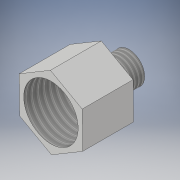
# Autodesk Inventor part: adapter
Saved by Autodesk Inventor 2018 (Build 220112000, 112)
## iProperties
Created: 2017-05-02
Part Number: adapter
Material: Generic
Document SubType Name: Modeling
Designer: gsegs
Density: 1 g/cm^3
Appearance: Default
Author: gsegs
Autodesk Inventor part; units mm, degrees
ref_plane "YZ Plane" through (0, 0, 0) normal (1, 0, 0) x (0, 1, 0)
ref_plane "XZ Plane" through (0, 0, 0) normal (0, 1, 0) x (-1, 0, 0)
ref_plane "XY Plane" through (0, 0, 0) normal (0, 0, 1) x (1, 0, 0)
sketch "Sketch1" plane through (0, 0, 0) normal (0, 0, 1) x (1, 0, 0)
  line L0 (21.8129, 13.019) -> (22.1812, -12.381)
  line L1 (22.1812, -12.381) -> (0.3684, -25.4)
  line L2 (0.3684, -25.4) -> (-21.8129, -13.019)
  line L3 (-21.8129, -13.019) -> (-22.1812, 12.381)
  line L4 (-22.1812, 12.381) -> (-0.3684, 25.4)
  line L5 (-0.3684, 25.4) -> (21.8129, 13.019)
  point P0 (0, 0)
  point P1 (0, 0)
  dimension "d0" = 25.4
  dimension "d1" = 120
  constraints: 12 end point, 1 coincident, 13 other
  measures "d0" vertical distance of L2.end L3.end
  measures "d1" angle of L2 L3
extrude "Extrusion1" add sketch "Sketch1" along normal blind 35.56
sketch "Sketch2" plane through (0, 0, 35.56) normal (0, 0, 1) x (1, 0, 0)
  circle A0 centre (0, 0) radius 19.05
  dimension "d4" = 38.1
  constraints: 1 centre point, 1 coincident
  measures "d4" diameter of A0
extrude "Extrusion2" cut sketch "Sketch2" against normal blind 30.48
sketch "Sketch3" plane through (0, 0, 0) normal (0, 0, -1) x (-1, 0, 0)
  circle A0 centre (0, 0) radius 10.922
  dimension "d7" = 21.844
  constraints: 1 centre point, 1 coincident
  measures "d7" diameter of A0
extrude "Extrusion3" add sketch "Sketch3" along normal blind 19.05
thread "Thread1" size "7/8-9 UNC" class "2A" standard "ANSI Unified Screw Threads" full length
thread "Thread2" size "1 1/2-6 UNC" class "2B" standard "ANSI Unified Screw Threads" full length
body "Solid1"
